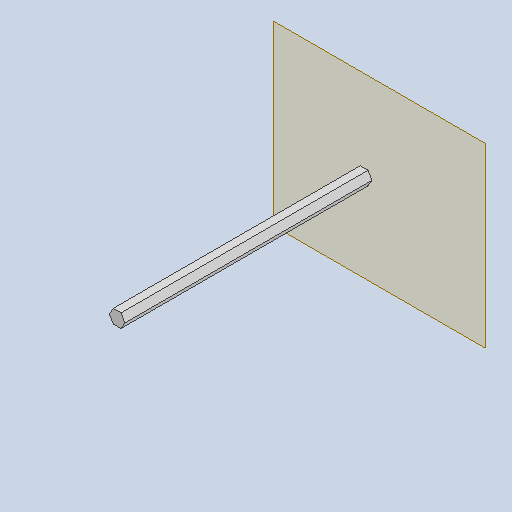
# Autodesk Inventor part: Eje_Salida
Saved by Autodesk Inventor 2022 (Build 260153000, 153)
## iProperties
Created: 2022-02-21
Part Number: Eje_Salida
Material: Generic
Document SubType Name: Modeling
Designer: katha
Density: 1 g/cm^3
Appearance: Default
Author: katha
Autodesk Inventor part; units mm, degrees
ref_plane "YZ Plane" through (0, 0, 0) normal (1, 0, 0) x (0, 1, 0)
ref_plane "XZ Plane" through (0, 0, 0) normal (0, 1, 0) x (-1, 0, 0)
ref_plane "XY Plane" through (0, 0, 0) normal (0, 0, 1) x (1, 0, 0)
ref_plane "Work Plane1" through (0, 0, 0) normal (0, 0, 1) x (1, 0, 0)
sketch "Sketch1" plane through (0, 0, 0) normal (0, 0, 1) x (1, 0, 0)
  line L0 (-37.6732, 2.8981) -> (-34.3268, 2.8981) projected
  line L1 (-39.3464, 0) -> (-37.6732, 2.8981) projected
  line L2 (-37.6732, -2.8981) -> (-39.3464, 0) projected
  line L3 (-34.3268, -2.8981) -> (-37.6732, -2.8981) projected
  line L4 (-32.6536, 0) -> (-34.3268, -2.8981) projected
  line L5 (-34.3268, 2.8981) -> (-32.6536, 0) projected
  line L6 (-34.5, 2.5981) -> (-37.5, 2.5981)
  line L7 (-37.5, 2.5981) -> (-39, 0)
  line L8 (-39, 0) -> (-37.5, -2.5981)
  line L9 (-37.5, -2.5981) -> (-34.5, -2.5981)
  line L10 (-34.5, -2.5981) -> (-33, 0)
  line L11 (-33, 0) -> (-34.5, 2.5981)
  point P0 (0, 0)
  dimension "d0" = 0.3
  constraints: 12 end point, 5 other
  measures "d0" distance between parallel lines of L0 L6
extrude "Extrusion1" add sketch "Sketch1" along normal blind 95 contours L11 L10 L9 L8 L7 L6
body "Solid1"
